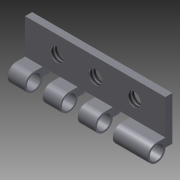
# Autodesk Inventor part: HingeP1
Saved by Autodesk Inventor 2012 (Build 160160000, 160)
## iProperties
Created: 2011-10-18
Part Number: HingeP1
Material: Default
Document SubType Name: Modeling
Designer: Smeet
Density: 1 g/cm^3
Author: Smeet
Autodesk Inventor part; units mm, degrees
ref_plane "YZ Plane" through (0, 0, 0) normal (1, 0, 0) x (0, 1, 0)
ref_plane "XZ Plane" through (0, 0, 0) normal (0, 1, 0) x (-1, 0, 0)
ref_plane "XY Plane" through (0, 0, 0) normal (0, 0, 1) x (1, 0, 0)
sketch "Sketch1" plane through (0, 0, 0) normal (0, 0, 1) x (1, 0, 0)
  line L0 (-21.147, 7.3925) -> (29.653, 7.3925)
  line L1 (29.653, 7.3925) -> (29.653, -5.3075)
  line L2 (29.653, -5.3075) -> (-21.147, -5.3075)
  line L3 (-21.147, -5.3075) -> (-21.147, 7.3925)
  point P0 (0, 0)
  dimension "d0" = 50.8
  dimension "d1" = 12.7
  constraints: 8 end point, 2 parallel, 1 horizontal, 1 perpendicular
  measures "d0" distance of L0.start L0.end
  measures "d1" distance of L2.end L0.start
extrude "Extrusion1" add sketch "Sketch1" along normal blind 2.54
sketch "Sketch3" plane through (29.653, -5.3075, 0) normal (1, 0, 0) x (0, 0, -1)
  line L0 (-2.54, 0) -> (-8.89, 0)
  line L1 (-8.89, 0) -> (-8.89, -6.35)
  line L2 (-8.89, -6.35) -> (-2.54, -6.35)
  line L3 (-2.54, -6.35) -> (-2.54, 0)
  point P0 (0, 5.3075)
  dimension "d9" = 6.35
  dimension "d10" = 6.35
  constraints: 8 end point, 2 parallel, 1 horizontal, 1 perpendicular
  measures "d9" distance of L0.start L0.end
  measures "d10" distance of L0.end L1.end
extrude "Extrusion2" add sketch "Sketch3" against normal blind 50.8
fillet "Fillet1" radius 3.175 3 edges at (4.253, -5.3075, 8.89) (4.253, -11.6575, 8.89) (4.253, -11.6575, 2.54)
hole "Hole1" at (29.653, -8.4825, 5.715) direction (-1, 0, 0) diameter 5.08 end through all
sketch "Sketch4" plane through (-21.147, -5.3075, 2.54) normal (0, 1, 0) x (1, 0, 0)
  line L0 (50.8, 0) -> (0, 0) projected
  line L1 (0, 0) -> (0, -3.175) projected
  line L2 (6.35, 0) -> (12.7, 0)
  line L3 (12.7, 0) -> (12.7, -6.6787)
  line L4 (12.7, -6.6787) -> (6.35, -6.6787)
  line L5 (6.35, -6.6787) -> (6.35, 0)
  line L6 (19.05, 0) -> (25.4, 0)
  line L7 (25.4, 0) -> (25.4, -6.6787)
  line L8 (25.4, -6.6787) -> (19.05, -6.6787)
  line L9 (19.05, -6.6787) -> (19.05, 0)
  line L10 (31.75, 0) -> (38.1, 0)
  line L11 (38.1, 0) -> (38.1, -6.6787)
  line L12 (38.1, -6.6787) -> (31.75, -6.6787)
  line L13 (31.75, -6.6787) -> (31.75, 0)
  point P0 (21.147, 2.54)
  dimension "d23" = 6.35
  dimension "d24" = 6.35
  dimension "d25" = 6.35
  dimension "d26" = 6.35
  dimension "d27" = 6.35
  dimension "d28" = 6.35
  constraints: 24 end point, 6 parallel, 3 horizontal, 3 perpendicular, 1 point on line
  measures "d23" distance between parallel lines of L1 L5
  measures "d24" distance of L3.end L4.end
  measures "d25" distance of L7.end L9.start
  measures "d26" distance of L11.end L13.start
  measures "d27" distance between parallel lines of L9 L3
  measures "d28" distance between parallel lines of L7 L13
extrude "Extrusion3" cut sketch "Sketch4" against normal blind 12.7
hole "Hole2" at (-9.717, 1.0425, 2.54) direction (0, 0, -1) diameter 4.9784 end through all thread size "1/4-20 UNC" class "2B" standard "ANSI Unified Screw Threads"
hole "Hole3" at (18.223, 1.0425, 2.54) direction (0, 0, -1) diameter 4.9784 end through all thread size "1/4-20 UNC" class "2B" standard "ANSI Unified Screw Threads"
hole "Hole4" at (4.253, 1.0425, 2.54) direction (0, 0, -1) diameter 4.9784 end through all thread size "1/4-20 UNC" class "2B" standard "ANSI Unified Screw Threads"
sketch "Sketch5" plane through (29.653, -8.4825, 2.54) normal (0, 0, -1) x (-1, 0, 0)
  line L0 (12.7, 0) -> (12.7, 3.175) projected
  line L1 (0, 3.175) -> (12.7, 3.175) projected
  line L2 (0, 3.175) -> (12.7, 3.175)
  line L3 (12.7, 3.175) -> (12.7, 0)
  line L4 (12.7, 0) -> (0, 0)
  line L5 (0, 0) -> (0, 3.175)
  point P0 (29.653, 8.4825)
  constraints: 8 end point, 2 parallel, 1 horizontal, 1 perpendicular
sketch "Sketch6" plane through (10.603, -8.4825, 2.54) normal (0, 0, -1) x (-1, 0, 0)
  line L0 (0, 3.175) -> (0, 0) projected
  line L1 (6.35, 0) -> (0, 0) projected
  line L2 (0, 3.175) -> (6.35, 3.175)
  line L3 (6.35, 3.175) -> (6.35, 0)
  line L4 (6.35, 0) -> (0, 0)
  line L5 (0, 0) -> (0, 3.175)
  point P0 (10.603, 8.4825)
  constraints: 8 end point, 2 parallel, 1 horizontal, 1 perpendicular
sketch "Sketch7" plane through (-2.097, -8.4825, 2.54) normal (0, 0, -1) x (-1, 0, 0)
  line L0 (0, 3.175) -> (0, 0) projected
  line L1 (6.35, 0) -> (0, 0) projected
  line L2 (0, 3.175) -> (6.35, 3.175)
  line L3 (6.35, 3.175) -> (6.35, 0)
  line L4 (6.35, 0) -> (0, 0)
  line L5 (0, 0) -> (0, 3.175)
  point P0 (-2.097, 8.4825)
  constraints: 8 end point, 2 parallel, 1 horizontal, 1 perpendicular
sketch "Sketch8" plane through (-21.147, -8.4825, 2.54) normal (0, 0, -1) x (-1, 0, 0)
  line L0 (-6.35, 3.175) -> (-6.35, 0) projected
  line L1 (0, 0) -> (-6.35, 0) projected
  line L2 (-6.35, 3.175) -> (0, 3.175)
  line L3 (0, 3.175) -> (0, 0)
  line L4 (0, 0) -> (-6.35, 0)
  line L5 (-6.35, 0) -> (-6.35, 3.175)
  point P0 (-21.147, 8.4825)
  constraints: 8 end point, 2 parallel, 1 horizontal, 1 perpendicular
extrude "Extrusion4" add sketch "Sketch5" along normal blind 2.54
extrude "Extrusion5" add sketch "Sketch6" along normal blind 2.54
extrude "Extrusion6" add sketch "Sketch7" along normal blind 2.54
extrude "Extrusion7" add sketch "Sketch8" along normal blind 2.54
body "Solid1"
